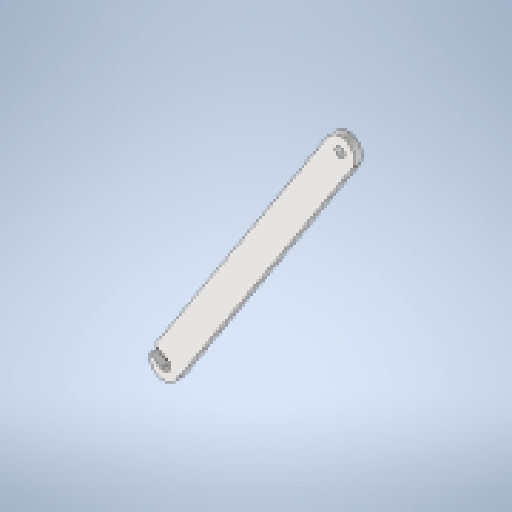
# Autodesk Inventor part: TheHandle
Saved by Autodesk Inventor 2025.1 (Build 291241000, 241)
## iProperties
Created: 2026-05-10
Part Number: TheHandle
Material: Generic
Document SubType Name: Modeling
Designer: User
Density: 1 g/cm^3
Appearance: Default
Author: User
Autodesk Inventor part; units mm, degrees
ref_plane "YZ Plane" through (0, 0, 0) normal (1, 0, 0) x (0, 1, 0)
ref_plane "XZ Plane" through (0, 0, 0) normal (0, 1, 0) x (-1, 0, 0)
ref_plane "XY Plane" through (0, 0, 0) normal (0, 0, 1) x (1, 0, 0)
sketch "Sketch1" plane through (0, 0, 0) normal (0, 0, 1) x (1, 0, 0)
  circle A0 centre (33.7394, 8.5) radius 2.5 projected
  circle A1 centre (-57.3324, -132.0207) radius 2.5 projected
  circle A2 centre (33.7394, 8.5) radius 7.5
  line L0 (40.0332, 4.421) -> (-51.0386, -136.0997)
  arc A3 (-64.7058, -130.6488) -> (-58.937, -134.5557) centre (33.7394, 8.5) ccw
  line L1 (27.4456, 12.579) -> (-61.9015, -125.2806)
  arc A4 (-64.7058, -130.6488) -> (-51.0386, -136.0997) centre (-57.3324, -132.0207) ccw
  arc A5 (-58.991, -134.5207) -> (-55.7273, -129.486) centre (-57.3324, -132.0207) ccw
  arc A6 (-61.9015, -125.2806) -> (-55.6742, -129.5204) centre (33.7394, 8.5) ccw
  point P0 (0, 0)
  dimension "d1" = 15
  constraints: 14 point on circle, 5 centre point, 4 coincident, 4 end point, 3 tangent
  measures "d1" diameter of A2
extrude "Extrusion1" add sketch "Sketch1" along normal blind 4 contours A2 | A2 L0 A4 A3 A5 A6 L1
body "Solid1"
